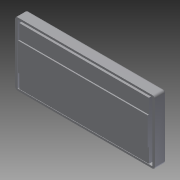
# Autodesk Inventor part: VLA-ST-60-12-0050WSlider
Saved by Autodesk Inventor 2011 SP1 (Build 150282100, 282)
## iProperties
Created: 2013-10-23
Part Number: VLA-ST-60-12-0050WSlider
Catalog Web Link: www.cadenas.de
Description: with Motor-S-
Vendor: THK
Document SubType Name: Modeling
Designer: PARTuser1
Manufacturer: THK
Density: 1 g/cm^3
Category: PARTsolutions
Company: THK
Title: VLA-ST-60-12-0050WSlider
Author: Cadenas PARTsolutions
PSOL_IDENT_0: {$CADENAS_DATA\23d-libs\thk\actuator\type_vla\slider_type_st\without_motor_2.prj},197 {VTYP=3D},{NB=
PSOL_IDENT_1: VLA-ST-60-12-0050WSlider},{LINA=VLA-ST-60-12-0050WSlider},{NN=with Motor-S},{DATE=01.03.2011 00:58:2
PSOL_IDENT_2: 1},{GEOMDATE=10.12.2007 12:18:00},{VERSION=},{LINEID=110},{LINESUBID=-1},{WBVAR=}  {NB=VLA-ST-60-12-
PSOL_IDENT_3: 0050WSlider},{LINA=VLA-ST-60-12-0050WSlider},{KT=DUMMY},{IDNR=},{SZ=VLA-ST-60-12-0050},{NDM=5.000},{
PSOL_IDENT_4: P=10.000},{L1=237.000},{SZ1=60}
CNS_NB: VLA-ST-60-12-0050WSlider
CNS_NBSYN: $SZ.WSlider
CNS_LINA: VLA-ST-60-12-0050WSlider
CNS_SZ: VLA-ST-60-12-0050
CNS_NDM: 5.000
CNS_P: 10.000
CNS_L1: 237.000
CNS_SZ1: 60
SUPPLIER: THK
ARTICLENO: VLA-ST-60-12-0050WSlider
BOMINFO: VLA-ST-60-12-0050WSlider
CREATOR: CADENAS GmbH
Autodesk Inventor part; units mm, degrees
sketch "Sketch_3" plane through (-0.5, 0, 0) normal (1, 0, 0) x (0, 0, -1)
  line L0 (-22.5, 22.4) -> (-22.5, 17.8)
  line L1 (-22.5, 17.8) -> (-11, 17.8)
  line L2 (-11, 17.8) -> (-11, 16.9)
  line L3 (-11, 16.9) -> (11, 16.9)
  line L4 (11, 16.9) -> (11, 17.8)
  line L5 (11, 17.8) -> (22.5, 17.8)
  line L6 (22.5, 17.8) -> (22.5, 22.4)
  arc A0 (22.5, 22.4) -> (21, 23.9) centre (21, 22.4) ccw
  line L7 (21, 23.9) -> (-21, 23.9)
  arc A1 (-21, 23.9) -> (-22.5, 22.4) centre (-21, 22.4) ccw
  constraints: 16 end point, 4 point on circle, 2 centre point
extrude "Extrusion1" add sketch "Sketch_3" along normal mid plane 102
sketch "Sketch_5" plane through (10.5, 0, 0) normal (1, 0, 0) x (0, 0, -1)
  line L0 (11.5, 18) -> (19.5, 18)
  line L1 (19.5, 18) -> (19.5, 28)
  line L2 (19.5, 28) -> (11.5, 28)
  line L3 (11.5, 28) -> (11.5, 18)
  constraints: 8 end point
extrude "Extrusion2" add sketch "Sketch_5" along normal blind 19.5
sketch "Sketch_6" plane through (-0.5, 0, 0) normal (1, 0, 0) x (0, 0, -1)
  line L0 (-25, 18.5) -> (-23.5, 18.5)
  line L1 (-23.5, 18.5) -> (-23.5, 26)
  line L2 (-23.5, 26) -> (23.5, 26)
  line L3 (23.5, 26) -> (23.5, 18.5)
  line L4 (23.5, 18.5) -> (25, 18.5)
  line L5 (25, 18.5) -> (25, 26)
  arc A0 (25, 26) -> (23.5, 27.5) centre (23.5, 26) ccw
  line L6 (23.5, 27.5) -> (-23.5, 27.5)
  arc A1 (-23.5, 27.5) -> (-25, 26) centre (-23.5, 26) ccw
  line L7 (-25, 26) -> (-25, 18.5)
  constraints: 16 end point, 4 point on circle, 2 centre point
extrude "Extrusion3" add sketch "Sketch_6" along normal mid plane 106
sketch "Sketch_7" plane through (0, 0, 0) normal (0, 0, 1) x (1, 0, 0)
  line L0 (-55.5, 18.5) -> (-53.5, 18.5)
  line L1 (-53.5, 18.5) -> (-53.5, 27.5)
  line L2 (-53.5, 27.5) -> (-54, 27.5)
  arc A0 (-54, 27.5) -> (-55.5, 26) centre (-54, 26) ccw
  line L3 (-55.5, 26) -> (-55.5, 18.5)
  constraints: 8 end point, 2 point on circle, 1 centre point
extrude "Extrusion4" add sketch "Sketch_7" along normal mid plane 46
sketch "Sketch_8" plane through (0, 0, 23) normal (0, 0, 1) x (1, 0, 0)
  line L0 (-53.5, 27.4142) -> (-53.5, 18.5)
  line L1 (-53.5, 18.5) -> (-55.5, 18.5)
  line L2 (-55.5, 18.5) -> (-55.5, 26)
  arc A0 (-53.5, 27.4142) -> (-55.5, 26) centre (-54, 26) ccw
  line L3 (-53.5, 27.4142) -> (-53.5, 18.5)
  constraints: 8 end point, 2 point on circle, 1 centre point
revolve "Revolution1" add sketch "Sketch_8" angle 90 about axis through (-53.5, 27.4142, 23) along (0, 1, 0)
sketch "Sketch_20" plane through (10.5, 0, 0) normal (1, 0, 0) x (0, 0, -1)
  line L0 (11.5, 18) -> (19.5, 18)
  line L1 (19.5, 18) -> (19.5, 28)
  line L2 (19.5, 28) -> (11.5, 28)
  line L3 (11.5, 28) -> (11.5, 18)
  constraints: 8 end point
extrude "Extrusion5" cut sketch "Sketch_20" along normal blind 0.1
sketch "Sketch_24" plane through (30, 0, 0) normal (1, 0, 0) x (0, 0, -1)
  line L0 (11.5, 18) -> (19.5, 18)
  line L1 (19.5, 18) -> (19.5, 28)
  line L2 (19.5, 28) -> (11.5, 28)
  line L3 (11.5, 28) -> (11.5, 18)
  constraints: 8 end point
extrude "Extrusion6" cut sketch "Sketch_24" along normal blind 0.1
sketch "Sketch_9" plane through (0, 0, -23) normal (0, 0, 1) x (1, 0, 0)
  line L0 (-53.5, 27.4142) -> (-53.5, 18.5)
  line L1 (-53.5, 18.5) -> (-55.5, 18.5)
  line L2 (-55.5, 18.5) -> (-55.5, 26)
  arc A0 (-53.5, 27.4142) -> (-55.5, 26) centre (-54, 26) ccw
  line L3 (-53.5, 27.4142) -> (-53.5, 18.5)
  constraints: 8 end point, 2 point on circle, 1 centre point
revolve "Revolution2" add sketch "Sketch_9" angle 90 about axis through (-53.5, 27.4142, -23) along (0, -1, 0)
sketch "Sketch_10" plane through (0, 0, 0) normal (0, 0, 1) x (1, 0, 0)
  line L0 (52.5, 18.5) -> (54.5, 18.5)
  line L1 (54.5, 18.5) -> (54.5, 26)
  arc A0 (54.5, 26) -> (53, 27.5) centre (53, 26) ccw
  line L2 (53, 27.5) -> (52.5, 27.5)
  line L3 (52.5, 27.5) -> (52.5, 18.5)
  constraints: 8 end point, 2 point on circle, 1 centre point
extrude "Extrusion7" add sketch "Sketch_10" along normal mid plane 46
sketch "Sketch_11" plane through (0, 0, -23) normal (0, 0, 1) x (1, 0, 0)
  line L0 (52.5, 18.5) -> (52.5, 27.4142)
  arc A0 (54.5, 26) -> (52.5, 27.4142) centre (53, 26) ccw
  line L1 (54.5, 26) -> (54.5, 18.5)
  line L2 (54.5, 18.5) -> (52.5, 18.5)
  line L3 (52.5, 18.5) -> (52.5, 27.4142)
  constraints: 8 end point, 2 point on circle, 1 centre point
revolve "Revolution3" add sketch "Sketch_11" angle 90 about axis through (52.5, 18.5, -23) along (0, 1, 0)
sketch "Sketch_12" plane through (0, 0, 23) normal (0, 0, 1) x (1, 0, 0)
  line L0 (52.5, 18.5) -> (52.5, 27.4142)
  arc A0 (54.5, 26) -> (52.5, 27.4142) centre (53, 26) ccw
  line L1 (54.5, 26) -> (54.5, 18.5)
  line L2 (54.5, 18.5) -> (52.5, 18.5)
  line L3 (52.5, 18.5) -> (52.5, 27.4142)
  constraints: 8 end point, 2 point on circle, 1 centre point
revolve "Revolution4" add sketch "Sketch_12" angle 90 about axis through (52.5, 18.5, 23) along (0, -1, 0)
sketch "Sketch_13" plane through (-30.1, 0, 0) normal (1, 0, 0) x (0, 0, -1)
  line L0 (11.5, 18) -> (19.5, 18)
  line L1 (19.5, 18) -> (19.5, 28)
  line L2 (19.5, 28) -> (11.5, 28)
  line L3 (11.5, 28) -> (11.5, 18)
  constraints: 8 end point
extrude "Extrusion8" cut sketch "Sketch_13" along normal blind 19.7
sketch "Sketch_14" plane through (-10.5, 0, 0) normal (1, 0, 0) x (0, 0, -1)
  line L0 (11.5, 18) -> (19.5, 18)
  line L1 (19.5, 18) -> (19.5, 28)
  line L2 (19.5, 28) -> (11.5, 28)
  line L3 (11.5, 28) -> (11.5, 18)
  constraints: 8 end point
extrude "Extrusion9" add sketch "Sketch_14" against normal blind 19.5
sketch "Sketch_15" plane through (10.4, 0, 0) normal (1, 0, 0) x (0, 0, -1)
  line L0 (-19.5, 18) -> (-11.5, 18)
  line L1 (-11.5, 18) -> (-11.5, 28)
  line L2 (-11.5, 28) -> (-19.5, 28)
  line L3 (-19.5, 28) -> (-19.5, 18)
  constraints: 8 end point
extrude "Extrusion10" cut sketch "Sketch_15" along normal blind 19.7
sketch "Sketch_16" plane through (10.5, 0, 0) normal (1, 0, 0) x (0, 0, -1)
  line L0 (-19.5, 18) -> (-11.5, 18)
  line L1 (-11.5, 18) -> (-11.5, 28)
  line L2 (-11.5, 28) -> (-19.5, 28)
  line L3 (-19.5, 28) -> (-19.5, 18)
  constraints: 8 end point
extrude "Extrusion11" add sketch "Sketch_16" along normal blind 19.5
sketch "Sketch_17" plane through (-30.1, 0, 0) normal (1, 0, 0) x (0, 0, -1)
  line L0 (-19.5, 18) -> (-11.5, 18)
  line L1 (-11.5, 18) -> (-11.5, 28)
  line L2 (-11.5, 28) -> (-19.5, 28)
  line L3 (-19.5, 28) -> (-19.5, 18)
  constraints: 8 end point
extrude "Extrusion12" cut sketch "Sketch_17" along normal blind 19.7
sketch "Sketch_18" plane through (-10.5, 0, 0) normal (1, 0, 0) x (0, 0, -1)
  line L0 (-19.5, 18) -> (-11.5, 18)
  line L1 (-11.5, 18) -> (-11.5, 28)
  line L2 (-11.5, 28) -> (-19.5, 28)
  line L3 (-19.5, 28) -> (-19.5, 18)
  constraints: 8 end point
extrude "Extrusion13" add sketch "Sketch_18" against normal blind 19.5
sketch "Sketch_19" plane through (25, 0, 0) normal (1, 0, 0) x (0, 0, -1)
  line L0 (15.5, 18) -> (15.5, 28)
  line L1 (15.5, 28) -> (18, 28)
  line L2 (18, 28) -> (17.567, 27.567)
  line L3 (17.567, 27.567) -> (17.567, 18.433)
  line L4 (17.567, 18.433) -> (18, 18)
  line L5 (18, 18) -> (15.5, 18)
  line L6 (15.5, 18) -> (15.5, 28)
  constraints: 14 end point
revolve "Revolution5" cut sketch "Sketch_19" angle 360 about axis through (25, 18, -15.5) along (0, -1, 0)
thread "Thread1" size "M5x0.8" class "6H" standard "ISO Metric profile" full length
sketch "Sketch_21" plane through (25, 0, 0) normal (1, 0, 0) x (0, 0, -1)
  line L0 (-15.5, 18) -> (-15.5, 28)
  line L1 (-15.5, 28) -> (-13, 28)
  line L2 (-13, 28) -> (-13.433, 27.567)
  line L3 (-13.433, 27.567) -> (-13.433, 18.433)
  line L4 (-13.433, 18.433) -> (-13, 18)
  line L5 (-13, 18) -> (-15.5, 18)
  line L6 (-15.5, 18) -> (-15.5, 28)
  constraints: 14 end point
revolve "Revolution6" cut sketch "Sketch_21" angle 360 about axis through (25, 18, 15.5) along (0, -1, 0)
thread "Thread2" size "M5x0.8" class "6H" standard "ISO Metric profile" full length
sketch "Sketch_23" plane through (-25, 0, 0) normal (1, 0, 0) x (0, 0, -1)
  line L0 (-15.5, 18) -> (-15.5, 28)
  line L1 (-15.5, 28) -> (-13, 28)
  line L2 (-13, 28) -> (-13.433, 27.567)
  line L3 (-13.433, 27.567) -> (-13.433, 18.433)
  line L4 (-13.433, 18.433) -> (-13, 18)
  line L5 (-13, 18) -> (-15.5, 18)
  line L6 (-15.5, 18) -> (-15.5, 28)
  constraints: 14 end point
revolve "Revolution7" cut sketch "Sketch_23" angle 360 about axis through (-25, 18, 15.5) along (0, -1, 0)
thread "Thread3" size "M5x0.8" class "6H" standard "ISO Metric profile" full length
sketch "Sketch_4" plane through (-25, 0, 0) normal (1, 0, 0) x (0, 0, -1)
  line L0 (15.5, 18) -> (15.5, 28)
  line L1 (15.5, 28) -> (18, 28)
  line L2 (18, 28) -> (17.567, 27.567)
  line L3 (17.567, 27.567) -> (17.567, 18.433)
  line L4 (17.567, 18.433) -> (18, 18)
  line L5 (18, 18) -> (15.5, 18)
  line L6 (15.5, 18) -> (15.5, 28)
  constraints: 14 end point
revolve "Revolution8" cut sketch "Sketch_4" angle 360 about axis through (-25, 18, -15.5) along (0, -1, 0)
thread "Thread4" size "M5x0.8" class "6H" standard "ISO Metric profile" full length
sketch "Sketch_27" plane through (0, 0, 0) normal (1, 0, 0) x (0, 1, 0)
  line L0 (26.3, -15.5) -> (27.5, -15.5)
  line L1 (27.5, -15.5) -> (27.5, -18.75)
  line L2 (27.5, -18.75) -> (26.3, -18.75)
  line L3 (26.3, -18.75) -> (26.3, -15.5)
  line L4 (26.3, -15.5) -> (27.5, -15.5)
  constraints: 10 end point
revolve "Revolution9" cut sketch "Sketch_27" angle 360 about axis through (0, 26.3, -15.5) along (0, -1, 0)
sketch "Sketch_28" plane through (0, 0, 0) normal (1, 0, 0) x (0, 1, 0)
  line L0 (26.3, -15.5) -> (27.3, -15.5)
  line L1 (27.3, -15.5) -> (27.3, -17.75)
  line L2 (27.3, -17.75) -> (26.3, -17.75)
  line L3 (26.3, -17.75) -> (26.3, -15.5)
  line L4 (26.3, -15.5) -> (27.3, -15.5)
  constraints: 10 end point
revolve "Revolution10" add sketch "Sketch_28" angle 360 about axis through (0, 26.3, -15.5) along (0, -1, 0)
sketch "Sketch_29" plane through (0, 0, 0) normal (1, 0, 0) x (0, 1, 0)
  line L0 (-50, -15.5) -> (50, -15.5)
  line L1 (26, -17.3) -> (26, -18.8)
  line L2 (26, -18.8) -> (27.3, -18.8)
  line L3 (27.3, -18.8) -> (26, -17.3)
  constraints: 8 end point
revolve "Revolution11" add sketch "Sketch_29" angle 360 about axis through (0, -50, -15.5) along (0, -1, 0)
sketch "Sketch_30" plane through (0, 27.3, 0) normal (0, 1, 0) x (1, 0, 0)
  line L0 (-0.8839, 14.9697) -> (-0.5303, 14.6161)
  line L1 (-0.5303, 14.6161) -> (0, 15.1464)
  line L2 (0, 15.1464) -> (0.5303, 14.6161)
  line L3 (0.5303, 14.6161) -> (0.8839, 14.9697)
  line L4 (0.8839, 14.9697) -> (0.3536, 15.5)
  line L5 (0.3536, 15.5) -> (0.8839, 16.0303)
  line L6 (0.8839, 16.0303) -> (0.5303, 16.3839)
  line L7 (0.5303, 16.3839) -> (0, 15.8536)
  line L8 (0, 15.8536) -> (-0.5303, 16.3839)
  line L9 (-0.5303, 16.3839) -> (-0.8839, 16.0303)
  line L10 (-0.8839, 16.0303) -> (-0.3536, 15.5)
  line L11 (-0.3536, 15.5) -> (-0.8839, 14.9697)
  constraints: 24 end point
extrude "Extrusion14" cut sketch "Sketch_30" against normal blind 2
sketch "Sketch_33" plane through (0, 0, 0) normal (1, 0, 0) x (0, 1, 0)
  line L0 (50, 15.5) -> (-50, 15.5)
  line L1 (26, 18.8) -> (26, 17.3)
  line L2 (26, 17.3) -> (27.3, 18.8)
  line L3 (27.3, 18.8) -> (26, 18.8)
  constraints: 8 end point
sketch "Sketch_31" plane through (0, 0, 0) normal (1, 0, 0) x (0, 1, 0)
  line L0 (26.3, 15.5) -> (27.5, 15.5)
  line L1 (27.5, 15.5) -> (27.5, 12.25)
  line L2 (27.5, 12.25) -> (26.3, 12.25)
  line L3 (26.3, 12.25) -> (26.3, 15.5)
  line L4 (26.3, 15.5) -> (27.5, 15.5)
  constraints: 10 end point
revolve "Revolution12" cut sketch "Sketch_31" angle 360 about axis through (0, 26.3, 15.5) along (0, -1, 0)
sketch "Sketch_32" plane through (0, 0, 0) normal (1, 0, 0) x (0, 1, 0)
  line L0 (26.3, 15.5) -> (27.3, 15.5)
  line L1 (27.3, 15.5) -> (27.3, 13.25)
  line L2 (27.3, 13.25) -> (26.3, 13.25)
  line L3 (26.3, 13.25) -> (26.3, 15.5)
  line L4 (26.3, 15.5) -> (27.3, 15.5)
  constraints: 10 end point
revolve "Revolution13" add sketch "Sketch_32" angle 360 about axis through (0, 26.3, 15.5) along (0, -1, 0)
revolve "Revolution14" add sketch "Sketch_33" angle 360 about axis through (0, 50, 15.5) along (0, 1, 0)
sketch "Sketch_34" plane through (0, 27.3, 0) normal (0, 1, 0) x (1, 0, 0)
  line L0 (-0.8839, -16.0303) -> (-0.5303, -16.3839)
  line L1 (-0.5303, -16.3839) -> (0, -15.8536)
  line L2 (0, -15.8536) -> (0.5303, -16.3839)
  line L3 (0.5303, -16.3839) -> (0.8839, -16.0303)
  line L4 (0.8839, -16.0303) -> (0.3536, -15.5)
  line L5 (0.3536, -15.5) -> (0.8839, -14.9697)
  line L6 (0.8839, -14.9697) -> (0.5303, -14.6161)
  line L7 (0.5303, -14.6161) -> (0, -15.1464)
  line L8 (0, -15.1464) -> (-0.5303, -14.6161)
  line L9 (-0.5303, -14.6161) -> (-0.8839, -14.9697)
  line L10 (-0.8839, -14.9697) -> (-0.3536, -15.5)
  line L11 (-0.3536, -15.5) -> (-0.8839, -16.0303)
  constraints: 24 end point
extrude "Extrusion15" cut sketch "Sketch_34" against normal blind 2
sketch "Sketch_1" plane through (0, 0, 15.5) normal (0, 0, 1) x (1, 0, 0)
  line L0 (-17, 18) -> (-17, 28)
  line L1 (-17, 28) -> (-15.5, 28)
  line L2 (-15.5, 28) -> (-15.5, 18)
  line L3 (-15.5, 18) -> (-17, 18)
  line L4 (-17, 18) -> (-17, 28)
  constraints: 10 end point
revolve "Revolution15" cut sketch "Sketch_1" angle 360 about axis through (-17, 18, 15.5) along (0, -1, 0)
sketch "Sketch_2" plane through (0, 0, 15.5) normal (0, 0, 1) x (1, 0, 0)
  line L0 (17, 18) -> (17, 28)
  line L1 (17, 28) -> (18.5, 28)
  line L2 (18.5, 28) -> (18.5, 18)
  line L3 (18.5, 18) -> (17, 18)
  line L4 (17, 18) -> (17, 28)
  constraints: 10 end point
revolve "Revolution16" cut sketch "Sketch_2" angle 360 about axis through (17, 18, 15.5) along (0, -1, 0)
sketch "Sketch_25" plane through (0, 0, -15.5) normal (0, 0, 1) x (1, 0, 0)
  line L0 (-17, 18) -> (-17, 28)
  line L1 (-17, 28) -> (-15.5, 28)
  line L2 (-15.5, 28) -> (-15.5, 18)
  line L3 (-15.5, 18) -> (-17, 18)
  line L4 (-17, 18) -> (-17, 28)
  constraints: 10 end point
revolve "Revolution17" cut sketch "Sketch_25" angle 360 about axis through (-17, 18, -15.5) along (0, -1, 0)
sketch "Sketch_26" plane through (0, 0, -15.5) normal (0, 0, 1) x (1, 0, 0)
  line L0 (17, 18) -> (17, 28)
  line L1 (17, 28) -> (18.5, 28)
  line L2 (18.5, 28) -> (18.5, 18)
  line L3 (18.5, 18) -> (17, 18)
  line L4 (17, 18) -> (17, 28)
  constraints: 10 end point
revolve "Revolution18" cut sketch "Sketch_26" angle 360 about axis through (17, 18, -15.5) along (0, -1, 0)
ref_plane "without_motor_s1_XY" through (0, 0, 0) normal (1, 0, 0) x (0, 0, -1)
ref_plane "without_motor_s1_YZ" through (0, 0, 0) normal (0, 0, -1) x (0, 1, 0)
ref_plane "without_motor_s1_ZX" through (0, 0, 0) normal (0, 1, 0) x (1, 0, 0)
body "Solid1"
